Autodesk Inventor part; units mm, degrees
(part 2 of 2)
sketch "Sketch14" plane through (0, 0, 0) normal (-1, 0, 0) x (0, 0, 1)
  line L0 (-34.1876, -176.7564) -> (25.2982, -176.7564) construction
  line L1 (25.2982, -176.7564) -> (25.2982, -164.2035) construction
  line L2 (25.2982, -164.2035) -> (-34.1876, -164.2035) construction
  line L3 (-34.1876, -164.2035) -> (-34.1876, -176.7564) construction
  line L4 (-27.0207, -184.7161) -> (-24.4518, -177.0961)
  line L5 (-24.4518, -177.0961) -> (-23.2045, -177.0961)
  line L6 (-23.2045, -177.0961) -> (-20.6357, -184.7161)
  line L7 (-20.6357, -184.7161) -> (-21.7039, -184.7161)
  line L8 (-21.7039, -184.7161) -> (-22.3955, -182.5857)
  line L9 (-22.3955, -182.5857) -> (-25.304, -182.5857)
  line L10 (-25.304, -182.5857) -> (-25.9956, -184.7161)
  line L11 (-25.9956, -184.7161) -> (-27.0207, -184.7161)
  line L12 (-22.6734, -181.7212) -> (-23.8529, -178.1335)
  line L13 (-23.8529, -178.1335) -> (-25.0261, -181.7212)
  line L14 (-25.0261, -181.7212) -> (-22.6734, -181.7212)
  line L15 (-14.016, -184.7161) -> (-15.3313, -184.7161)
  line L16 (-15.3313, -184.7161) -> (-17.7396, -181.6841)
  line L17 (-17.7396, -181.6841) -> (-18.9005, -181.6841)
  line L18 (-18.9005, -181.6841) -> (-18.9005, -184.7161)
  line L19 (-18.9005, -184.7161) -> (-19.9132, -184.7161)
  line L20 (-19.9132, -184.7161) -> (-19.9132, -177.0961)
  line L21 (-19.9132, -177.0961) -> (-17.9495, -177.0961)
  spline S0 degree 2 poles (-17.9495, -177.0961) (-17.295, -177.0961) (-16.4119, -177.2381) (-16.0106, -177.4974) knots 0 0 0 1 2 2 2
  spline S1 degree 2 poles (-16.0106, -177.4974) (-15.6092, -177.7568) (-15.1461, -178.5657) (-15.1461, -179.1647) knots 0 0 0 1 2 2 2
  spline S2 degree 2 poles (-15.1461, -179.1647) (-15.1461, -179.9983) (-15.9982, -181.1284) (-16.7269, -181.4001) knots 0 0 0 1 2 2 2
  line L22 (-16.7269, -181.4001) -> (-14.016, -184.7161)
  spline S3 degree 2 poles (-16.202, -179.245) (-16.202, -178.9115) (-16.4366, -178.399) (-16.6836, -178.2323) knots 0 0 0 1 2 2 2
  spline S4 degree 2 poles (-16.6836, -178.2323) (-16.8998, -178.0902) (-17.474, -177.9729) (-17.8939, -177.9729) knots 0 0 0 1 2 2 2
  line L23 (-17.8939, -177.9729) -> (-18.9005, -177.9729)
  line L24 (-18.9005, -177.9729) -> (-18.9005, -180.8381)
  line L25 (-18.9005, -180.8381) -> (-18.0113, -180.8381)
  spline S5 degree 2 poles (-18.0113, -180.8381) (-17.5728, -180.8381) (-16.8751, -180.6838) (-16.6342, -180.4429) knots 0 0 0 1 2 2 2
  spline S6 degree 2 poles (-16.6342, -180.4429) (-16.4119, -180.233) (-16.202, -179.6402) (-16.202, -179.245) knots 0 0 0 1 2 2 2
  line L26 (-11.6325, -184.7161) -> (-11.6325, -177.9976)
  line L27 (-11.6325, -177.9976) -> (-14.1889, -177.9976)
  line L28 (-14.1889, -177.9976) -> (-14.1889, -177.0961)
  line L29 (-14.1889, -177.0961) -> (-8.0633, -177.0961)
  line L30 (-8.0633, -177.0961) -> (-8.0633, -177.9976)
  line L31 (-8.0633, -177.9976) -> (-10.6197, -177.9976)
  line L32 (-10.6197, -177.9976) -> (-10.6197, -184.7161)
  line L33 (-10.6197, -184.7161) -> (-11.6325, -184.7161)
  spline S7 degree 2 poles (-5.1672, -184.8519) (-5.9946, -184.8519) (-7.1555, -184.5061) (-7.6681, -184.2591) knots 0 0 0 1 2 2 2
  line L34 (-7.6681, -184.2591) -> (-7.6681, -182.987)
  line L35 (-7.6681, -182.987) -> (-7.594, -182.987)
  spline S8 degree 2 poles (-7.594, -182.987) (-7.0938, -183.4564) (-5.8279, -183.9751) (-5.2413, -183.9751) knots 0 0 0 1 2 2 2
  spline S9 degree 2 poles (-5.2413, -183.9751) (-4.4015, -183.9751) (-3.5432, -183.2773) (-3.5432, -182.703) knots 0 0 0 1 2 2 2
  spline S10 degree 2 poles (-3.5432, -182.703) (-3.5432, -182.246) (-3.9939, -181.6779) (-4.4818, -181.5359) knots 0 0 0 1 2 2 2
  spline S11 degree 2 poles (-4.4818, -181.5359) (-4.8337, -181.4371) (-5.4204, -181.3013) (-5.8588, -181.1901) knots 0 0 0 1 2 2 2
  spline S12 degree 2 poles (-5.8588, -181.1901) (-6.254, -181.0851) (-6.8777, -180.7702) (-7.1185, -180.517) knots 0 0 0 1 2 2 2
  spline S13 degree 2 poles (-7.1185, -180.517) (-7.3532, -180.2639) (-7.6125, -179.5846) (-7.6125, -179.14) knots 0 0 0 1 2 2 2
  spline S14 degree 2 poles (-7.6125, -179.14) (-7.6125, -178.2137) (-6.1675, -176.9602) (-5.0499, -176.9602) knots 0 0 0 1 2 2 2
  spline S15 degree 2 poles (-5.0499, -176.9602) (-4.4077, -176.9602) (-3.2714, -177.2134) (-2.7836, -177.4542) knots 0 0 0 1 2 2 2
  line L36 (-2.7836, -177.4542) -> (-2.7836, -178.6645)
  line L37 (-2.7836, -178.6645) -> (-2.8577, -178.6645)
  spline S16 degree 2 poles (-2.8577, -178.6645) (-3.222, -178.3311) (-4.3583, -177.8371) (-4.9819, -177.8371) knots 0 0 0 1 2 2 2
  spline S17 degree 2 poles (-4.9819, -177.8371) (-5.6859, -177.8371) (-6.5566, -178.4978) (-6.5566, -179.035) knots 0 0 0 1 2 2 2
  spline S18 degree 2 poles (-6.5566, -179.035) (-6.5566, -179.5167) (-6.044, -180.091) (-5.5624, -180.2206) knots 0 0 0 1 2 2 2
  spline S19 degree 2 poles (-5.5624, -180.2206) (-5.2413, -180.3071) (-4.3089, -180.5294) (-4.0001, -180.622) knots 0 0 0 1 2 2 2
  spline S20 degree 2 poles (-4.0001, -180.622) (-3.2159, -180.8628) (-2.4872, -181.8323) (-2.4872, -182.5424) knots 0 0 0 1 2 2 2
  spline S21 degree 2 poles (-2.4872, -182.5424) (-2.4872, -182.9932) (-2.8515, -183.8577) (-3.1788, -184.1603) knots 0 0 0 1 2 2 2
  spline S22 degree 2 poles (-3.1788, -184.1603) (-3.5432, -184.4938) (-4.4694, -184.8519) (-5.1672, -184.8519) knots 0 0 0 1 2 2 2
  line L38 (1.119, -181.8447) -> (-1.7647, -181.8447)
  line L39 (-1.7647, -181.8447) -> (-1.7647, -180.9184)
  line L40 (-1.7647, -180.9184) -> (1.119, -180.9184)
  line L41 (1.119, -180.9184) -> (1.119, -181.8447)
  line L42 (6.763, -184.7161) -> (2.3478, -184.7161)
  line L43 (2.3478, -184.7161) -> (2.3478, -177.0961)
  line L44 (2.3478, -177.0961) -> (3.3605, -177.0961)
  line L45 (3.3605, -177.0961) -> (3.3605, -183.8145)
  line L46 (3.3605, -183.8145) -> (6.763, -183.8145)
  line L47 (6.763, -183.8145) -> (6.763, -184.7161)
  spline S23 degree 2 poles (10.6718, -184.1109) (10.5545, -184.1974) (10.1593, -184.5061) (9.974, -184.5987) knots 0 0 0 1 2 2 2
  spline S24 degree 2 poles (9.974, -184.5987) (9.7208, -184.7346) (9.2454, -184.8766) (8.8131, -184.8766) knots 0 0 0 1 2 2 2
  spline S25 degree 2 poles (8.8131, -184.8766) (8.4611, -184.8766) (7.8251, -184.6111) (7.5843, -184.3703) knots 0 0 0 1 2 2 2
  spline S26 degree 2 poles (7.5843, -184.3703) (7.3558, -184.1356) (7.0779, -183.444) (7.0779, -183.0611) knots 0 0 0 1 2 2 2
  spline S27 degree 2 poles (7.0779, -183.0611) (7.0779, -182.4683) (7.5781, -181.6285) (8.1215, -181.3877) knots 0 0 0 1 2 2 2
  spline S28 degree 2 poles (8.1215, -181.3877) (8.6032, -181.1654) (9.9123, -180.9987) (10.6718, -180.9555) knots 0 0 0 1 2 2 2
  line L48 (10.6718, -180.9555) -> (10.6718, -180.7702)
  spline S29 degree 2 poles (10.6718, -180.7702) (10.6718, -180.4368) (10.468, -180.023) (10.2828, -179.9057) knots 0 0 0 1 2 2 2
  spline S30 degree 2 poles (10.2828, -179.9057) (10.0975, -179.7884) (9.5665, -179.7143) (9.2824, -179.7143) knots 0 0 0 1 2 2 2
  spline S31 degree 2 poles (9.2824, -179.7143) (8.949, -179.7143) (8.0474, -179.9119) (7.5966, -180.1033) knots 0 0 0 1 2 2 2
  line L49 (7.5966, -180.1033) -> (7.541, -180.1033)
  line L50 (7.541, -180.1033) -> (7.541, -179.1215)
  spline S32 degree 2 poles (7.541, -179.1215) (7.8066, -179.0474) (8.8008, -178.8621) (9.2886, -178.8621) knots 0 0 0 1 2 2 2
  spline S33 degree 2 poles (9.2886, -178.8621) (9.8814, -178.8621) (10.6903, -179.0474) (11.0114, -179.2882) knots 0 0 0 1 2 2 2
  spline S34 degree 2 poles (11.0114, -179.2882) (11.3263, -179.5229) (11.6351, -180.27) (11.6351, -180.8073) knots 0 0 0 1 2 2 2
  line L51 (11.6351, -180.8073) -> (11.6351, -184.7161)
  line L52 (11.6351, -184.7161) -> (10.6718, -184.7161)
  line L53 (10.6718, -184.7161) -> (10.6718, -184.1109)
  line L54 (10.6718, -183.3082) -> (10.6718, -181.7212)
  spline S35 degree 2 poles (10.6718, -181.7212) (10.326, -181.752) (9.2824, -181.857) (8.9551, -181.9558) knots 0 0 0 1 2 2 2
  spline S36 degree 2 poles (8.9551, -181.9558) (8.5723, -182.0731) (8.0721, -182.561) (8.0721, -182.9932) knots 0 0 0 1 2 2 2
  spline S37 degree 2 poles (8.0721, -182.9932) (8.0721, -183.4872) (8.6279, -183.9874) (9.1589, -183.9874) knots 0 0 0 1 2 2 2
  spline S38 degree 2 poles (9.1589, -183.9874) (9.6097, -183.9874) (10.3507, -183.5984) (10.6718, -183.3082) knots 0 0 0 1 2 2 2
  spline S39 degree 2 poles (17.7793, -181.7644) (17.7793, -183.1661) (16.4208, -184.8766) (15.3957, -184.8766) knots 0 0 0 1 2 2 2
  spline S40 degree 2 poles (15.3957, -184.8766) (14.9326, -184.8766) (14.2718, -184.6481) (13.9507, -184.4505) knots 0 0 0 1 2 2 2
  line L55 (13.9507, -184.4505) -> (13.889, -184.7161)
  line L56 (13.889, -184.7161) -> (12.9874, -184.7161)
  line L57 (12.9874, -184.7161) -> (12.9874, -176.7564)
  line L58 (12.9874, -176.7564) -> (13.9507, -176.7564)
  line L59 (13.9507, -176.7564) -> (13.9507, -179.597)
  spline S41 degree 2 poles (13.9507, -179.597) (14.3151, -179.2697) (15.161, -178.8374) (15.6983, -178.8374) knots 0 0 0 1 2 2 2
  spline S42 degree 2 poles (15.6983, -178.8374) (16.6678, -178.8374) (17.7793, -180.3874) (17.7793, -181.7644) knots 0 0 0 1 2 2 2
  spline S43 degree 2 poles (16.7851, -181.8385) (16.7851, -180.8134) (16.1614, -179.7513) (15.4698, -179.7513) knots 0 0 0 1 2 2 2
  spline S44 degree 2 poles (15.4698, -179.7513) (15.0808, -179.7513) (14.278, -180.1218) (13.9507, -180.4059) knots 0 0 0 1 2 2 2
  line L60 (13.9507, -180.4059) -> (13.9507, -183.6848)
  spline S45 degree 2 poles (13.9507, -183.6848) (14.3151, -183.8639) (14.877, -184.0121) (15.2104, -184.0121) knots 0 0 0 1 2 2 2
  spline S46 degree 2 poles (15.2104, -184.0121) (15.9453, -184.0121) (16.7851, -182.9685) (16.7851, -181.8385) knots 0 0 0 1 2 2 2
  point P0 (0, 0)
  constraints: 2 other
emboss "Emboss2" sketch "Sketch14" operation cut depth 2.54 direction (1, 0, 0)
sketch "Sketch15" plane through (0, -201.0841, 48.4212) normal (0, 0, 1) x (1, 0, 0)
  line L0 (21.59, 0) -> (21.59, 248.666) projected
  line L1 (17.272, 161.671) -> (21.59, 161.671)
  line L2 (21.59, 161.671) -> (21.59, 175.387)
  line L3 (21.59, 175.387) -> (17.272, 175.387)
  line L4 (17.272, 175.387) -> (17.272, 161.671)
  line L5 (21.59, 251.841) -> (0, 251.841) projected
  line L6 (0, -3.175) -> (21.59, -3.175) projected
  point P0 (0, 201.0841)
  point P1 (19.431, 175.387)
  dimension "d78" = 13.716
  dimension "d79" = 4.318
  dimension "d216" = 164.846
  constraints: 8 end point, 2 parallel, 1 horizontal, 1 midpoint, 1 perpendicular, 1 point on line
  measures "d78" distance of L3.end L1.start
  measures "d79" distance between parallel lines of L0 L4
  measures "d216" distance between parallel lines of L6 L1
extrude "Extrusion9" cut sketch "Sketch15" against normal blind 8.89
sketch "Sketch18" plane through (0, -204.2591, -57.6238) normal (0, -1, 0) x (1, 0, 0)
  line L0 (21.59, 50.9016) -> (21.59, 60.9092)
  line L1 (21.59, 60.9092) -> (20.3708, 60.9092)
  line L2 (20.3708, 60.9092) -> (18.6182, 58.9092)
  line L3 (18.6182, 52.9016) -> (18.6182, 58.9092)
  line L4 (21.59, 106.045) -> (0, 106.045) projected
  line L5 (21.59, 102.87) -> (21.59, 0) projected
  line L6 (21.59, 50.9016) -> (20.3708, 50.9016)
  line L7 (20.3708, 50.9016) -> (18.6182, 52.9016)
  point P0 (20.9804, 60.9092)
  dimension "d91" = 1.2192
  dimension "d92" = 2
  dimension "d94" = 6.0076
  dimension "d95" = 10.0076
  dimension "d98" = 1.7526
  dimension "d99" = 0
  dimension "d165" = 45.1358
  constraints: 12 end point, 1 horizontal, 1 midpoint
  measures "d91" distance of L0.end L1.end
  measures "d92" vertical distance of L1.end L2.end
  measures "d94" distance of L3.start L2.end
  measures "d95" distance of L0.start L0.end
  measures "d98" distance from line of L1.end L3
  measures "d99" distance between parallel lines of L5 L0
  measures "d165" distance from line of L4 point (20.98, 60.909)
extrude "Extrusion10" cut sketch "Sketch18" against normal blind 6.35
sketch "Sketch19" plane through (0, 13.9785, -4.7779) normal (-1, 0, 0) x (0, 0, 1)
  arc A0 (-48.6469, 32.7145) -> (-49.2899, 28.3675) centre (-49.9249, 30.6825) ccw projected
  circle A1 centre (-49.9249, 30.6825) radius 4.5085
  arc A2 (45.8251, 32.7145) -> (46.4681, 28.3675) centre (47.1031, 30.6825) ccw projected
  circle A3 centre (47.1031, 30.6825) radius 4.5085
  circle A4 centre (-49.9249, -212.1415) radius 2.4005 projected
  circle A5 centre (-49.9249, -212.1415) radius 4.5085
  arc A6 (45.1674, -213.5612) -> (46.4681, -209.8265) centre (47.1031, -212.1415) ccw projected
  circle A7 centre (47.1031, -212.1415) radius 4.5085
  circle A8 centre (-43.9559, -64.8215) radius 4.5085
  circle A9 centre (-43.9559, -64.8215) radius 2.4005 projected
  circle A10 centre (41.1341, -64.8215) radius 4.5085
  circle A11 centre (41.1341, -64.8215) radius 2.4005 projected
  point P0 (0, 0)
  point P1 (-43.5669, 32.7145)
  point P2 (48.9872, -224.0625)
  point P3 (-44.5909, 33.7355)
  point P4 (46.8491, 29.6614)
  point P5 (-46.1229, 32.7145)
  point P6 (45.8251, -214.1735)
  point P7 (49.0081, -200.7677)
  dimension "d110" = 9.017
  dimension "d111" = 9.017
  dimension "d112" = 9.017
  dimension "d113" = 9.017
  dimension "d120" = 9.017
  dimension "d121" = 0
  dimension "d122" = 0
  dimension "d123" = 9.017
  dimension "d124" = 0
  dimension "d125" = 0
  constraints: 6 centre point, 4 coincident, 1 other
  measures "d110" diameter of A1
  measures "d111" diameter of A3
  measures "d112" diameter of A5
  measures "d113" diameter of A7
  measures "d120" diameter of A8
  measures "d121" distance of A9.centre A8.centre
  measures "d122" distance of A9.centre A8.centre
  measures "d123" diameter of A10
  measures "d124" distance of A11.centre A10.centre
  measures "d125" distance of A11.centre A10.centre
extrude "Extrusion11" cut sketch "Sketch19" against normal blind 5 contours A1 | A3 | A4 | A5 | A7 | A8 | A9 | A10 | A11
sketch "Sketch20" plane through (0, -204.2591, -57.6238) normal (0, -1, 0) x (1, 0, 0)
  circle A0 centre (19.558, 73.0374) radius 2.032
  line L0 (21.59, 106.045) -> (0, 106.045) projected
  line L1 (21.59, 102.87) -> (21.59, 60.9092) projected
  point P0 (0, 57.6238)
  dimension "d126" = 4.064
  dimension "d127" = 33.0076
  dimension "d128" = 2.032
  constraints: 1 centre point
  measures "d126" diameter of A0
  measures "d127" distance from line of L0 A0.centre
  measures "d128" distance from line of L1 A0.centre
extrude "Extrusion12" cut sketch "Sketch20" against normal blind 13.97
sketch "Sketch21" plane through (6.35, 0, 0) normal (1, 0, 0) x (0, 0, -1)
  line L0 (46.8288, -56.4311) -> (46.8288, -70.6551)
  line L1 (45.0508, -56.0234) -> (45.0508, -45.6876)
  line L2 (46.7824, -42.8597) -> (49.932, -41.2521)
  line L3 (51.293, -39.9128) -> (51.9088, -38.7527)
  line L4 (46.7824, -58.8513) -> (49.932, -60.4589)
  line L5 (51.293, -61.7982) -> (51.9088, -62.9583)
  arc A0 (51.293, -61.7982) -> (49.932, -60.4589) centre (48.4886, -63.2868) ccw
  arc A1 (45.0508, -56.0234) -> (46.7824, -58.8513) centre (48.2258, -56.0234) ccw
  arc A2 (49.932, -41.2521) -> (51.293, -39.9128) centre (48.4886, -38.4241) ccw
  arc A3 (46.7824, -42.8597) -> (45.0508, -45.6876) centre (48.2258, -45.6876) ccw
  line L6 (51.9088, -38.7527) -> (51.9088, -62.9583)
  line L7 (51.9088, -38.7527) -> (51.9088, -62.9583)
  line L8 (51.9088, -194.7341) -> (51.9088, 41.2319) projected
  line L9 (51.9088, 41.2319) -> (51.9088, -194.7341) projected
  line L10 (51.9088, -38.7527) -> (51.9088, -62.9583)
  circle A4 centre (48.7338, -50.8431) radius 2.4005 projected
  circle A5 centre (48.7338, -50.8431) radius 2.4005
  line L11 (-39.5312, -194.7341) -> (-39.5312, 41.2319)
  line L12 (-39.5312, -70.6551) -> (-39.5312, -56.4311)
  line L13 (-32.6732, -45.7067) -> (-32.6732, -56.0428)
  line L14 (-34.4046, -58.8706) -> (-37.5542, -60.4785)
  line L15 (-38.9053, -61.7996) -> (-39.5312, -62.9605)
  line L16 (-34.4046, -42.8789) -> (-37.5542, -41.271)
  line L17 (-38.9385, -39.8868) -> (-39.5312, -38.7257)
  arc A6 (-37.5542, -60.4785) -> (-38.9053, -61.7996) centre (-36.1106, -63.3063) ccw
  arc A7 (-34.4046, -58.8706) -> (-32.6732, -56.0428) centre (-35.8482, -56.0428) ccw
  arc A8 (-32.6732, -45.7067) -> (-34.4046, -42.8789) centre (-35.8482, -45.7067) ccw
  arc A9 (-38.9385, -39.8868) -> (-37.5542, -41.271) centre (-36.1106, -38.4432) ccw
  line L18 (-39.5312, -38.7257) -> (-39.5312, -62.9605)
  line L19 (-39.5312, 41.2319) -> (-39.5312, -194.7341) projected
  circle A10 centre (-36.3562, -50.8431) radius 2.4005
  point P0 (0, 0)
  point P1 (-37.853, -70.6551)
  point P2 (43.3998, -52.8751)
  point P3 (50.8236, -40.797)
  point P4 (46.8288, -57.8659)
  point P5 (46.8288, -56.4311)
  point P6 (46.8288, -57.8659)
  point P7 (49.3688, -48.5281)
  point P8 (49.3688, -53.1581)
  point P9 (49.3688, 43.6399)
  point P10 (49.3688, 50.7569)
  point P11 (-38.4357, -60.9285)
  point P12 (-38.4706, -40.8032)
  dimension "d215" = 0
  dimension "d181" = 145
  dimension "d182" = 145
  dimension "d183" = 117.04
  dimension "d184" = 117.04
  dimension "d185" = 3.175
  dimension "d187" = 3.175
  dimension "d188" = 3.1496
  dimension "d189" = 2.0443
  dimension "d190" = 3.1496
  dimension "d209" = 24.2056
  dimension "d219" = 12.0904
  dimension "d227" = 6.858
  dimension "d228" = 117.044
  dimension "d229" = 117.044
  dimension "d230" = 2.032
  dimension "d231" = 3.175
  dimension "d232" = 3.1496
  dimension "d233" = 3.1496
  dimension "d234" = 24.2348
  dimension "d236" = 12.1174
  dimension "d237" = 0
  constraints: 32 end point, 16 point on circle, 16 tangent, 10 centre point, 10 point on line, 6 equal radius, 2 coincident, 2 parallel, 2 vertical, 1 perpendicular, 6 other
  measures "d181" angle of L2 L3
  measures "d182" angle of L5 L4
  measures "d183" angle of L4 L1
  measures "d184" angle of L1 L2
  measures "d185" radius of A0
  measures "d187" radius of A2
  measures "d188" horizontal distance of L2.start L2.end
  measures "d189" vertical distance of L3.end point (50.824, -40.797)
  measures "d190" horizontal distance of L4.start L4.end
  measures "d209" distance of L5.end L3.end
  measures "d219" vertical distance of A4.centre L10.start
  measures "d227" distance between parallel lines of L11 L13
  measures "d228" angle of L14 L13
  measures "d229" angle of L16 L13
  measures "d230" vertical distance of point (-38.436, -60.928) L15.end
  measures "d231" radius of A6
  measures "d232" horizontal distance of L14.start L14.end
  measures "d233" horizontal distance of L16.start L16.end
  measures "d234" distance of L15.end L18.start
  measures "d236" vertical distance of point (-36.356, -50.843) L18.start
  measures "d237" distance between parallel lines of L19 L11
extrude "Extrusion13" add sketch "Sketch21" along normal blind 10.16
sketch "Sketch22" plane through (0, -204.2591, -57.6238) normal (0, -1, 0) x (1, 0, 0)
  line L0 (21.59, 73.0374) -> (21.59, 50.9016) projected
  line L1 (13.97, 9.525) -> (21.59, 9.525)
  line L2 (21.59, 9.525) -> (21.59, 93.345)
  line L3 (21.59, 93.345) -> (13.97, 93.345)
  line L4 (13.97, 93.345) -> (13.97, 9.525)
  line L5 (21.59, 106.045) -> (0, 106.045) projected
  line L6 (0, -3.175) -> (21.59, -3.175) projected
  line L7 (10.4902, 45.3136) -> (13.97, 45.3136)
  line L8 (13.97, 45.3136) -> (13.97, 56.3372)
  line L9 (13.97, 56.3372) -> (10.4902, 56.3372)
  line L10 (10.4902, 56.3372) -> (10.4902, 45.3136)
  line L11 (21.59, 56.3372) -> (20.1405, 56.3372) projected
  line L12 (20.1405, 45.3136) -> (21.59, 45.3136) projected
  line L13 (18.1102, 54.0203) -> (18.1102, 47.6305) projected
  point P0 (0, 57.6238)
  point P1 (21.59, 96.139)
  point P2 (17.78, 93.345)
  point P3 (17.78, 9.525)
  point P4 (20.8653, 56.3372)
  point P5 (12.2301, 56.3372)
  point P6 (20.8653, 45.3136)
  point P7 (10.4902, 50.8254)
  dimension "d191" = 12.7
  dimension "d192" = 12.7
  dimension "d193" = 0
  dimension "d194" = 0
  dimension "d195" = 7.62
  dimension "d203" = 7.62
  constraints: 16 end point, 6 midpoint, 4 parallel, 2 horizontal, 2 perpendicular, 2 point on line
  measures "d191" distance from line of L5 point (17.78, 93.345)
  measures "d192" distance from line of L6 point (17.78, 9.525)
  measures "d193" vertical distance of point (20.865, 56.337) point (12.23, 56.337)
  measures "d194" distance from line of point (20.865, 45.314) L7
  measures "d195" distance from line of L13 point (10.49, 50.825)
  measures "d203" distance between parallel lines of L2 L4
extrude "Extrusion14" cut sketch "Sketch22" against normal blind 7.62
fillet "Fillet7" radius 0.762 4 edges at (10.4902, -201.0841, -1.2866) (10.4902, -201.0841, -12.3102) (13.97, -201.0841, -12.3102) (13.97, -201.0841, -1.2866)
fillet "Fillet8" radius 0.762 11 edges at (13.7468, -204.2591, -1.0634) (12.2301, -204.2591, -1.2866) (10.7134, -204.2591, -1.5098) (10.4902, -204.2591, -6.7984) (10.7134, -204.2591, -12.087) (12.2301, -204.2591, -12.3102) (13.7468, -204.2591, -12.5334) (13.97, -204.2591, -30.5855) (13.97, -204.2591, 17.5983) (17.78, -204.2591, -48.0988) (17.78, -204.2591, 35.7212)
sketch "Sketch23" plane through (17.78, 46.6929, 9.0512) normal (1, 0, 0) x (0, 0, -1)
  line L0 (0, 4.064) -> (57.15, 4.064) projected
  line L1 (0, 0) -> (57.15, 0) projected
  line L2 (56.7066, 4.064) -> (39.37, 4.064)
  line L3 (39.37, 4.064) -> (39.37, 0)
  line L4 (39.37, 0) -> (56.7066, 0)
  line L5 (0, 0) -> (0, 4.064) projected
  line L6 (56.7066, 4.064) -> (56.7066, 0)
  point P0 (9.0512, -46.6929)
  point P1 (0, 2.032)
  point P2 (39.37, 4.064)
  point P3 (56.7066, 0)
  point P4 (56.7066, 4.064)
  dimension "d221" = 39.37
  constraints: 8 end point, 2 perpendicular, 1 horizontal, 1 midpoint, 1 parallel, 1 point on line
  measures "d221" distance from line of point (0, 2.032) L3
extrude "Extrusion15" add sketch "Sketch23" along normal blind 8.89 contours L0 L6 L1 L3
fillet "Fillet9" radius 0.508 7 edges at (19.685, 50.7569, 9.0512) (17.78, 50.7569, -10.6338) (22.225, 50.7569, -30.3188) (26.67, 50.7569, -38.9871) (19.431, -25.6971, 48.4212) (17.272, -32.5551, 48.4212) (19.431, -39.4131, 48.4212)
sketch "Sketch24" plane through (17.78, 46.6929, 9.0512) normal (1, 0, 0) x (0, 0, -1)
  line L0 (0, 4.064) -> (0, 0) projected
  line L1 (39.37, 0) -> (39.37, 4.064) projected
  line L2 (0, 0) -> (39.37, 0)
  line L3 (39.37, 0) -> (39.37, 2.032)
  line L4 (39.37, 2.032) -> (0, 2.032)
  line L5 (0, 2.032) -> (0, 0)
  point P0 (9.0512, -46.6929)
  point P1 (0, 2.032)
  dimension "d240" = 2.032
  constraints: 8 end point, 2 parallel, 1 horizontal, 1 midpoint, 1 perpendicular
  measures "d240" distance between parallel lines of L2 L4
extrude "Extrusion16" add sketch "Sketch24" along normal blind 0.508
sketch "Sketch25" plane through (17.78, 46.6929, -48.0988) normal (1, 0, 0) x (0, 0, -1)
  line L0 (-0.4434, 4.064) -> (-0.4434, 3.556) projected
  line L1 (-0.4434, 4.064) -> (0, 4.064)
  line L2 (0, 4.064) -> (0, 0)
  line L3 (0, 0) -> (-0.4434, 0)
  line L4 (-0.4434, 0) -> (-0.4434, 4.064)
  point P0 (-48.0988, -46.6929)
  constraints: 8 end point, 2 parallel, 1 horizontal, 1 perpendicular
extrude "Extrusion17" add sketch "Sketch25" along normal blind 3.81
body "Solid1"
